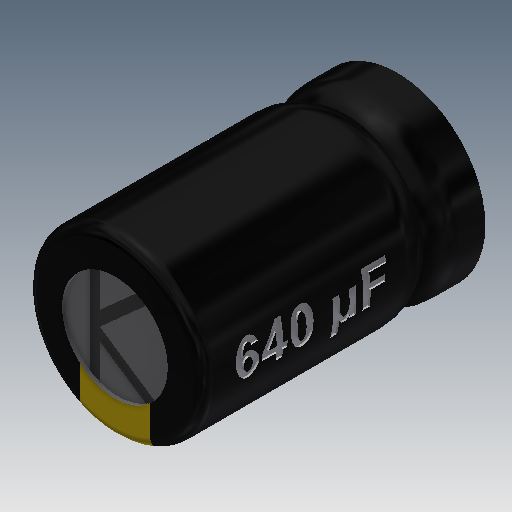
# Autodesk Inventor part: config - capasitor 640 μF
Saved by Autodesk Inventor 2019.1 (Build 231200000, 200)
## iProperties
Company: Autodesk Asia Pte. Ltd.
Created: 2005-12-06
Part Number: config - capasitor 640 μF
Document SubType Name: Modeling
Designer: Simon.Ng@autodesk.com
Stock Number: config - capasitor 640 μF
Density: 1 g/cm^3
Material: Generic
Mass: 0.154062 g
Surface Area: 1.66494 cm^2
Volume: 0.154062 cm^3
Appearance: Glossy - Black
Title: PC Demo
Author: Simon.Ng@autodesk.com
Autodesk Inventor part; units mm, degrees
ref_plane "YZ Plane" through (0, 0, 0) normal (1, 0, 0) x (0, 1, 0)
ref_plane "XZ Plane" through (0, 0, 0) normal (0, 1, 0) x (-1, 0, 0)
ref_plane "XY Plane" through (0, 0, 0) normal (0, 0, 1) x (1, 0, 0)
sketch "Sketch1" plane through (0, 0, 0) normal (0, 0, 1) x (1, 0, 0)
  line L0 (0, 4) -> (0, -3) construction
  line L1 (-3, 0) -> (4, 0) construction
  circle A0 centre (0, 0) radius 2.5
  dimension "d0" = 5
  constraints: 2 point on line, 1 centre point
  measures "d0" diameter of A0
extrude "Extrusion1" add sketch "Sketch1" along normal blind 8
sketch "Sketch6" plane through (0, 0, 0) normal (1, 0, 0) x (0, 1, 0)
  line L0 (0, 10.4) -> (0, -0.8) projected
  line L1 (2.5, 0) -> (2.5, 8) projected
  line L2 (2.5, 2.25) -> (2.5, 0.75)
  line L3 (2.5, 1.5) -> (2.25, 1.5) construction
  line L4 (-2.5, 0) -> (2.5, 0) construction
  arc A0 (2.25, 1.5) -> (2.5, 2.25) centre (1.25, 2.25) ccw
  arc A1 (2.5, 0.75) -> (2.25, 1.5) centre (1.25, 0.75) ccw
  point P0 (0, 0)
  dimension "d16" = 1.5
  dimension "d17" = 1.5
  dimension "d18" = 0.25
  constraints: 4 end point, 4 point on circle, 2 centre point, 2 point on line, 2 tangent, 1 collinear, 1 horizontal, 1 midpoint
  measures "d16" distance of L2.start L2.end
  measures "d17" distance between parallel lines of L4 L3
  measures "d18" distance of L3.start L3.end
revolve "Revolution1" cut sketch "Sketch6" angle 360 about axis through (0, 0, 0) along (0, 0, -1)
sketch "Sketch2" plane through (0, 0, 8) normal (0, 0, 1) x (1, 0, 0)
  circle A0 centre (0, 0) radius 2.5 projected
  circle A1 centre (0, 0) radius 1.5
  dimension "d3" = 1
  constraints: 1 centre point, 1 coincident
  measures "d3" radial gap between concentric circles of A1 A0
extrude "Extrusion2" cut sketch "Sketch2" against normal blind 0.1 contours A1
sketch "Sketch3" plane through (0, 0, 7.9) normal (0, 0, 1) x (1, 0, 0)
  line L0 (-0.8063, 1.4052) -> (-0.5247, 1.4052)
  line L1 (-0.5247, 1.4052) -> (-0.5247, -1.4052)
  line L2 (-0.5247, -1.4052) -> (-0.8063, -1.4052)
  line L3 (-0.8063, -1.4052) -> (-0.8063, 1.4052)
  line L4 (-0.5247, -0.0512) -> (-0.7319, 0.1806)
  line L5 (-0.7319, 0.1806) -> (0.679, 1.442)
  line L6 (0.679, 1.442) -> (0.8862, 1.2102)
  line L7 (0.8862, 1.2102) -> (-0.5247, -0.0512)
  line L8 (-0.5247, -0.0512) -> (-0.6915, -0.2996)
  line L9 (-0.6915, -0.2996) -> (0.8602, -1.3417)
  line L10 (0.8602, -1.3417) -> (1.027, -1.0933)
  line L11 (1.027, -1.0933) -> (-0.5247, -0.0512)
  circle A0 centre (0, 0) radius 1.5 projected
  constraints: 24 end point, 6 parallel, 4 point on circle, 3 perpendicular, 1 horizontal, 1 point on line
extrude "Extrusion3" cut sketch "Sketch3" against normal blind 0.05 contours L0 A0 L3 | L1 L5 L4 L8 L9 A0 L3 | L5 A0 L7 L1 | L1 L4 L5 | L5 L6 A0 | A0 L2 L3 | L11 A0 L9 L1 | L1 L9 L8 | L10 L9 A0
fillet "Fillet1" radius 0.3 1 edges at (-2.5, 0, 8)
sketch "Sketch5" plane through (0, 0, 8) normal (0, 0, 1) x (1, 0, 0)
  circle A0 centre (0, 0) radius 1.5 projected
  circle A1 centre (0, 0) radius 2.5 projected
  line L0 (0, -3) -> (0, 4) projected
  line L1 (-1, -1.118) -> (-1, -3)
  line L2 (-1, -3) -> (1, -3)
  line L3 (1, -3) -> (1, -1.118)
  point P0 (0, -2.5)
  point P1 (0, -2.5)
  dimension "d20" = 2
  dimension "d21" = 0.5
  constraints: 6 end point, 2 parallel, 2 point on circle, 1 coincident, 1 perpendicular, 1 point on line, 1 vertical alignment, 2 other
  measures "d20" distance of L1.end L2.end
  measures "d21" distance from line of L2 point (0, -2.5)
split_face "Split1"
ref_plane "Work Plane1" through (10, 0, 0) normal (1, 0, 0) x (0, 1, 0)
sketch "Sketch4" plane through (10, 0, 0) normal (1, 0, 0) x (0, 0, -1)
  line L0 (-7.1279, 0.625) -> (8.4803, 0.625) construction
  line L1 (8.4803, 0.625) -> (8.4803, -3.2142) construction
  line L2 (8.4803, -3.2142) -> (-7.1279, -3.2142) construction
  line L3 (-7.1279, -3.2142) -> (-7.1279, 0.625) construction
  line L4 (-6.4191, 0.3765) -> (-6.6043, 0.3559)
  spline S0 degree 3 poles (-6.6043, 0.3559) (-6.6112, 0.4131) (-6.6683, 0.4672) (-6.7141, 0.4672) knots 0 0 0 0 1 1 1 1
  spline S1 degree 3 poles (-6.7141, 0.4672) (-6.775, 0.4672) (-6.8589, 0.3582) (-6.8695, 0.1859) knots 0 0 0 0 1 1 1 1
  spline S2 degree 2 poles (-6.8695, 0.1859) (-6.7987, 0.2705) (-6.6919, 0.2705) knots 0 0 0 1 1 1
  spline S3 degree 3 poles (-6.6919, 0.2705) (-6.5723, 0.2705) (-6.4008, 0.0876) (-6.4008, -0.0564) knots 0 0 0 0 1 1 1 1
  spline S4 degree 3 poles (-6.4008, -0.0564) (-6.4008, -0.2104) (-6.5807, -0.3956) (-6.7217, -0.3956) knots 0 0 0 0 1 1 1 1
  spline S5 degree 3 poles (-6.7217, -0.3956) (-6.8734, -0.3956) (-7.0685, -0.1601) (-7.0685, 0.1074) knots 0 0 0 0 1 1 1 1
  spline S6 degree 3 poles (-7.0685, 0.1074) (-7.0685, 0.3826) (-6.865, 0.625) (-6.7026, 0.625) knots 0 0 0 0 1 1 1 1
  spline S7 degree 3 poles (-6.7026, 0.625) (-6.5891, 0.625) (-6.4397, 0.4977) (-6.4191, 0.3765) knots 0 0 0 0 1 1 1 1
  spline S8 degree 3 poles (-6.8535, -0.0412) (-6.8535, -0.1349) (-6.7674, -0.2363) (-6.7125, -0.2363) knots 0 0 0 0 1 1 1 1
  spline S9 degree 3 poles (-6.7125, -0.2363) (-6.6592, -0.2363) (-6.5883, -0.1532) (-6.5883, -0.0587) knots 0 0 0 0 1 1 1 1
  spline S10 degree 3 poles (-6.5883, -0.0587) (-6.5883, 0.0388) (-6.6645, 0.1295) (-6.7217, 0.1295) knots 0 0 0 0 1 1 1 1
  spline S11 degree 3 poles (-6.7217, 0.1295) (-6.7773, 0.1295) (-6.8535, 0.0426) (-6.8535, -0.0412) knots 0 0 0 0 1 1 1 1
  line L5 (-5.916, -0.3788) -> (-5.916, -0.1776)
  line L6 (-5.916, -0.1776) -> (-6.3253, -0.1776)
  line L7 (-6.3253, -0.1776) -> (-6.3253, -0.0107)
  line L8 (-6.3253, -0.0107) -> (-5.8916, 0.625)
  line L9 (-5.8916, 0.625) -> (-5.7308, 0.625)
  line L10 (-5.7308, 0.625) -> (-5.7308, -0.0099)
  line L11 (-5.7308, -0.0099) -> (-5.6066, -0.0099)
  line L12 (-5.6066, -0.0099) -> (-5.6066, -0.1776)
  line L13 (-5.6066, -0.1776) -> (-5.7308, -0.1776)
  line L14 (-5.7308, -0.1776) -> (-5.7308, -0.3788)
  line L15 (-5.7308, -0.3788) -> (-5.916, -0.3788)
  line L16 (-5.916, -0.0099) -> (-5.916, 0.3323)
  line L17 (-5.916, 0.3323) -> (-6.1462, -0.0099)
  line L18 (-6.1462, -0.0099) -> (-5.916, -0.0099)
  spline S12 degree 2 poles (-5.1912, 0.625) (-5.0456, 0.625) (-4.9641, 0.5213) knots 0 0 0 1 1 1
  spline S13 degree 2 poles (-4.9641, 0.5213) (-4.8665, 0.3986) (-4.8665, 0.1143) knots 0 0 0 1 1 1
  spline S14 degree 2 poles (-4.8665, 0.1143) (-4.8665, -0.1692) (-4.9648, -0.2935) knots 0 0 0 1 1 1
  spline S15 degree 2 poles (-4.9648, -0.2935) (-5.0456, -0.3956) (-5.1912, -0.3956) knots 0 0 0 1 1 1
  spline S16 degree 3 poles (-5.1912, -0.3956) (-5.3375, -0.3956) (-5.5159, -0.1715) (-5.5159, 0.1166) knots 0 0 0 0 1 1 1 1
  spline S17 degree 2 poles (-5.5159, 0.1166) (-5.5159, 0.3986) (-5.4176, 0.5228) knots 0 0 0 1 1 1
  spline S18 degree 2 poles (-5.4176, 0.5228) (-5.3368, 0.625) (-5.1912, 0.625) knots 0 0 0 1 1 1
  spline S19 degree 3 poles (-5.1912, 0.4657) (-5.2262, 0.4657) (-5.2804, 0.4215) (-5.2956, 0.3643) knots 0 0 0 0 1 1 1 1
  spline S20 degree 2 poles (-5.2956, 0.3643) (-5.3154, 0.2904) (-5.3154, 0.1143) knots 0 0 0 1 1 1
  spline S21 degree 4 poles (-5.3154, 0.1143) (-5.3154, -0.061) (-5.2796, -0.1929) (-5.2262, -0.2363) (-5.1912, -0.2363) knots 0 0 0 0 0 1 1 1 1 1
  spline S22 degree 3 poles (-5.1912, -0.2363) (-5.1561, -0.2363) (-5.102, -0.1921) (-5.0868, -0.1349) knots 0 0 0 0 1 1 1 1
  spline S23 degree 2 poles (-5.0868, -0.1349) (-5.0669, -0.061) (-5.0669, 0.1143) knots 0 0 0 1 1 1
  spline S24 degree 4 poles (-5.0669, 0.1143) (-5.0669, 0.2904) (-5.1028, 0.4215) (-5.1561, 0.4657) (-5.1912, 0.4657) knots 0 0 0 0 0 1 1 1 1 1
  line L19 (-4.3116, 0.346) -> (-4.1195, 0.346)
  line L20 (-4.1195, 0.346) -> (-4.1195, 0.0167)
  spline S25 degree 4 poles (-4.1195, 0.0167) (-4.1195, -0.0755) (-4.1005, -0.1792) (-4.0334, -0.2432) (-3.9862, -0.2432) knots 0 0 0 0 0 1 1 1 1 1
  spline S26 degree 4 poles (-3.9862, -0.2432) (-3.9374, -0.2432) (-3.8665, -0.1761) (-3.8459, -0.0808) (-3.8459, 0.0144) knots 0 0 0 0 0 1 1 1 1 1
  line L21 (-3.8459, 0.0144) -> (-3.8459, 0.346)
  line L22 (-3.8459, 0.346) -> (-3.6538, 0.346)
  line L23 (-3.6538, 0.346) -> (-3.6538, -0.3788)
  line L24 (-3.6538, -0.3788) -> (-3.8307, -0.3788)
  line L25 (-3.8307, -0.3788) -> (-3.8307, -0.2912)
  spline S27 degree 2 poles (-3.8307, -0.2912) (-3.884, -0.3949) (-3.9762, -0.3949) knots 0 0 0 1 1 1
  spline S28 degree 2 poles (-3.9762, -0.3949) (-4.0738, -0.3949) (-4.1195, -0.2912) knots 0 0 0 1 1 1
  line L26 (-4.1195, -0.2912) -> (-4.1195, -0.6548)
  line L27 (-4.1195, -0.6548) -> (-4.3116, -0.6548)
  line L28 (-4.3116, -0.6548) -> (-4.3116, 0.346)
  line L29 (-3.4534, -0.3788) -> (-3.4534, 0.6212)
  line L30 (-3.4534, 0.6212) -> (-2.7666, 0.6212)
  line L31 (-2.7666, 0.6212) -> (-2.7666, 0.4519)
  line L32 (-2.7666, 0.4519) -> (-3.2514, 0.4519)
  line L33 (-3.2514, 0.4519) -> (-3.2514, 0.2157)
  line L34 (-3.2514, 0.2157) -> (-2.833, 0.2157)
  line L35 (-2.833, 0.2157) -> (-2.833, 0.0465)
  line L36 (-2.833, 0.0465) -> (-3.2514, 0.0465)
  line L37 (-3.2514, 0.0465) -> (-3.2514, -0.3788)
  line L38 (-3.2514, -0.3788) -> (-3.4534, -0.3788)
  constraints: 2 other
emboss "Emboss1" sketch "Sketch4" operation cut depth 0.05 direction (1, 0, 0) wrap yes faces at (-0.3066, 2.4811, 4.0667) (-0.3066, 2.4811, 4.0667) (-0.3066, 2.4811, 4.0667) (-0.3066, 2.4811, 0.5) (-0.3066, 2.4811, 0.5) (-0.3066, 2.4811, 0.5) (-0.3066, 2.4811, 0.5) (-0.3066, 2.4811, 4.0667)
body "Solid1"
